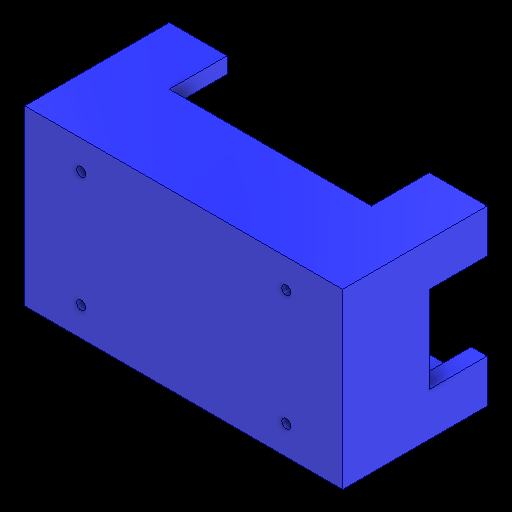
# Autodesk Inventor part: magnet_holder
Saved by Autodesk Inventor 2026.1 (Build 301233000, 233)
## iProperties
Created: 2025-09-30
Part Number: magnet_holder
Material: PC/ABS Plastic
Document SubType Name: Modeling
Designer: drago
Density: 1.1 g/cm^3
Appearance: Blue - Wall Paint - Glossy
Mass: 119.67 g
Surface Area: 407.663 cm^2
Volume: 108.791 cm^3
Author: drago
Autodesk Inventor part; units mm, degrees
ref_plane "YZ Plane" through (0, 0, 0) normal (1, 0, 0) x (0, 1, 0)
ref_plane "XZ Plane" through (0, 0, 0) normal (0, 1, 0) x (-1, 0, 0)
ref_plane "XY Plane" through (0, 0, 0) normal (0, 0, 1) x (1, 0, 0)
sketch "Sketch1" plane through (0, 0, 0) normal (0, 0, 1) x (1, 0, 0)
  line L0 (55, -30) -> (-55, -30)
  line L1 (-55, -30) -> (-55, 30)
  line L2 (-55, 30) -> (55, 30)
  line L3 (55, 30) -> (55, -30)
  line L4 (49.5, -24.5) -> (-49.5, -24.5)
  line L5 (-49.5, -24.5) -> (-49.5, 24.5)
  line L6 (-49.5, 24.5) -> (49.5, 24.5)
  line L7 (49.5, 24.5) -> (49.5, -24.5)
  line L8 (55, 0) -> (-55, 0) construction
  line L9 (0, -30) -> (0, 30) construction
  line L10 (-35, 30) -> (-35, 24.5)
  line L11 (-55, 15) -> (-49.5, 15)
  line L12 (35, -24.5) -> (35, -30)
  line L13 (49.5, -15) -> (55, -15)
  line L14 (-35, -24.5) -> (-35, -30)
  line L15 (-55, -15) -> (-49.5, -15)
  line L16 (35, 30) -> (35, 24.5)
  line L17 (49.5, 15) -> (55, 15)
  line L18 (-52.25, 27.25) -> (52.25, 27.25) construction
  line L19 (52.25, 27.25) -> (52.25, -27.25) construction
  line L20 (52.25, -27.25) -> (-52.25, -27.25) construction
  line L21 (-52.25, -27.25) -> (-52.25, 27.25) construction
  line L22 (-52.25, 27.25) -> (52.25, -27.25) construction
  line L23 (52.25, 27.25) -> (-52.25, -27.25) construction
  point P0 (0, 0)
  point P1 (-35.5, 20)
  point P2 (35.5, 20)
  point P3 (35.5, -20)
  point P4 (-35.5, -20)
  dimension "d0" = 110
  dimension "d1" = 60
  dimension "d2" = 99
  dimension "d3" = 49
  dimension "d4" = 15
  dimension "d5" = 20
  dimension "d6" = 40
  dimension "d7" = 71
  constraints: 48 end point, 16 point on line, 12 perpendicular, 6 midpoint, 6 parallel, 4 coincident, 4 collinear, 3 horizontal, 3 symmetric about line, 7 other
  measures "d0" distance of L1.end L2.end
  measures "d1" distance between parallel lines of L0 L2
  measures "d2" distance of L5.end L6.end
  measures "d3" distance of L4.end L5.end
  measures "d4" distance between parallel lines of L0 L13
  measures "d5" distance between parallel lines of L3 L12
  measures "d6" distance of point (35.5, 20) point (35.5, -20)
  measures "d7" distance of point (35.5, -20) point (-35.5, -20)
extrude "Extrusion1" add sketch "Sketch1" against normal blind 40 contours L0 L12 L4 L7 L13 L3 | L0 L1 L15 L5 L4 L14 | L17 L7 L6 L16 L2 L3 | L1 L2 L10 L6 L5 L11
extrude "Extrusion2" add sketch "Sketch1" along normal blind 10
hole "Hole1" at (-35.5, 20, 0) at (35.5, 20, 0) at (35.5, -20, 0) at (-35.5, -20, 0) direction (0, 0, 1) diameter 3.2 end through all counterbore diameter 6 counterbore depth 5
extrude "Extrusion8" add sketch "Sketch1" against normal blind 20 contours L0 L14 L4 L12 | L13 L7 L17 L3 | L1 L11 L5 L15 | L16 L6 L10 L2
equation "\"epsilon\" = 0"
body "Solid2"
